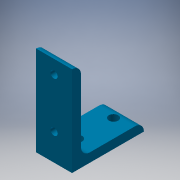
# Autodesk Inventor part: support L
Saved by Autodesk Inventor 2017 SP1 (Build 210196100, 196)
## iProperties
Created: 2018-01-20
Part Number: support L
Material: Aluminum 6061
Document SubType Name: Modeling
Designer: Ben
Density: 2.7 g/cm^3
Appearance: Sky Blue Medium
Mass: 44.5475 g
Surface Area: 72.0032 cm^2
Volume: 16.4991 cm^3
Author: Ben
Autodesk Inventor part; units mm, degrees
ref_plane "YZ Plane" through (0, 0, 0) normal (1, 0, 0) x (0, 1, 0)
ref_plane "XZ Plane" through (0, 0, 0) normal (0, 1, 0) x (-1, 0, 0)
ref_plane "XY Plane" through (0, 0, 0) normal (0, 0, 1) x (1, 0, 0)
sketch "Sketch1" plane through (0, 0, 0) normal (1, 0, 0) x (0, 1, 0)
  line L0 (0, 0) -> (63.5, 0)
  line L1 (0, 0) -> (0, -50.8)
  arc A0 (0, -50.8) -> (6.35, -44.45) centre (0, -44.45) ccw
  arc A1 (57.15, -6.35) -> (63.5, 0) centre (57.15, 0) ccw
  line L2 (57.15, -6.35) -> (12.7, -6.35)
  line L3 (6.35, -44.45) -> (6.35, -12.7)
  arc A2 (12.7, -6.35) -> (6.35, -12.7) centre (12.7, -12.7) ccw
  dimension "d0" = 6.35
  dimension "d1" = 63.5
  dimension "d16" = 50.8
  constraints: 8 end point, 6 point on circle, 4 tangent, 3 centre point, 2 equal radius, 2 horizontal, 2 line through centre, 2 vertical
  measures "d0" distance between parallel lines of L1 L3
  measures "d1" distance of L0.start L0.end
  measures "d16" distance of L0.start L1.end
extrude "Extrusion1" add sketch "Sketch1" along normal mid plane 25.4
sketch "Sketch2" plane through (-12.7, 0, 0) normal (0, 0, 1) x (1, 0, 0)
  line L0 (25.4, 6.35) -> (0, 6.35) projected
  line L1 (25.4, 6.35) -> (0, 6.35) projected
  line L2 (25.4, 6.35) -> (0, 6.35) construction
  line L3 (12.7, 6.35) -> (12.7, 63.5) construction
  line L4 (25.4, 63.5) -> (0, 63.5) construction
  circle A0 centre (12.7, 19.05) radius 2.54
  circle A1 centre (12.7, 53.975) radius 2.54
  point P0 (12.7, 0)
  dimension "d4" = 5.08
  dimension "d5" = 12.7
  dimension "d6" = 9.525
  constraints: 2 centre point, 2 end point, 2 midpoint, 2 point on line, 1 equal radius
  measures "d4" diameter of A0
  measures "d5" distance from line of L0 A0.centre
  measures "d6" distance from line of L4 A1.centre
extrude "Extrusion2" cut sketch "Sketch2" against normal through all
sketch "Sketch3" plane through (-12.7, 0, -50.8) normal (0, -1, 0) x (1, 0, 0)
  line L0 (25.4, 44.45) -> (0, 44.45) projected
  line L1 (25.4, 0) -> (0, 0) construction
  line L2 (12.7, 0) -> (12.7, 44.45) construction
  circle A0 centre (12.7, 34.163) radius 3.302
  circle A1 centre (12.7, 8.763) radius 3.302
  point P0 (12.7, 50.8)
  dimension "d9" = 6.604
  dimension "d14" = 16.637
  dimension "d15" = 25.4
  constraints: 2 centre point, 2 end point, 2 midpoint, 2 point on line, 1 equal radius
  measures "d9" diameter of A0
  measures "d14" distance of point (12.7, 50.8) A0.centre
  measures "d15" distance of A0.centre A1.centre
extrude "Extrusion3" cut sketch "Sketch3" against normal through all
body "Solid1"
